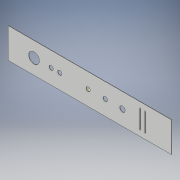
# Autodesk Inventor part: Faceplate
Saved by Autodesk Inventor 2017 (Build 210142000, 142)
## iProperties
Created: 2017-03-30
Part Number: Faceplate
Material: Generic
Document SubType Name: Sheet Metal
Designer: plumbj
Density: 1 g/cm^3
Appearance: Default
Sheet Metal Rule: Default
Author: plumbj
Autodesk Inventor part; units mm, degrees
ref_plane "YZ Plane" through (0, 0, 0) normal (1, 0, 0) x (0, 1, 0)
ref_plane "XZ Plane" through (0, 0, 0) normal (0, 1, 0) x (-1, 0, 0)
ref_plane "XY Plane" through (0, 0, 0) normal (0, 0, 1) x (1, 0, 0)
sketch "Sketch1" plane through (0, 0, 0) normal (0, 0, 1) x (1, 0, 0)
  line L0 (-241.3, -44.45) -> (241.3, -44.45)
  line L1 (241.3, -44.45) -> (241.3, 44.45)
  line L2 (241.3, 44.45) -> (-241.3, 44.45)
  line L3 (-241.3, 44.45) -> (-241.3, -44.45)
  point P0 (0, 0)
  dimension "d0" = 482.6
  dimension "d1" = 88.9
  dimension "d62" = 44.45
  dimension "d63" = 241.3
  constraints: 8 end point, 2 parallel, 1 horizontal, 1 perpendicular
  measures "d0" distance of L2.end L1.end
  measures "d1" distance of L1.end L0.end
  measures "d62" distance from line of L2 point (0, 0)
  measures "d63" distance from line of point (0, 0) L1
extrude "Extrusion1" add sketch "Sketch1" along normal blind 1.1113
sketch "Sketch3" plane through (0, 0, 1.1113) normal (0, 0, 1) x (1, 0, 0)
  point P0 (0, 0)
sketch "Sketch4" plane through (0, 0, 1.1113) normal (0, 0, 1) x (1, 0, 0)
  line L0 (147.5, 26.0031) -> (150.1, 26.0031)
  line L1 (150.1, 26.0031) -> (150.1, -25.9969)
  line L2 (150.1, -25.9969) -> (147.5, -25.9969)
  line L3 (147.5, -25.9969) -> (147.5, 26.0031)
  line L4 (162.5, 26.0031) -> (165.1, 26.0031)
  line L5 (165.1, 26.0031) -> (165.1, -25.9969)
  line L6 (165.1, -25.9969) -> (162.5, -25.9969)
  line L7 (162.5, -25.9969) -> (162.5, 26.0031)
  line L8 (-241.3, -44.45) -> (241.3, -44.45) projected
  line L9 (241.3, -44.45) -> (241.3, 44.45) projected
  circle A0 centre (-114.3, 0) radius 6.2484
  circle A1 centre (-88.9, 0) radius 6.2484
  circle A2 centre (-4.9, 0) radius 6.2484
  circle A3 centre (45.9, 0) radius 6.5
  circle A4 centre (96.7, 0) radius 8
  line L10 (241.3, 44.45) -> (-241.3, 44.45) projected
  line L11 (-241.3, -44.45) -> (241.3, -44.45) projected
  line L12 (241.3, -44.45) -> (241.3, 44.45) projected
  line L13 (241.3, 44.45) -> (-241.3, 44.45) projected
  line L14 (-241.3, 44.45) -> (-241.3, -44.45) projected
  circle A5 centre (163.8, 28.0031) radius 1.05
  circle A6 centre (163.8, -27.9969) radius 1.05
  circle A7 centre (148.8, 28.0031) radius 1.05
  circle A8 centre (148.8, -27.9969) radius 1.05
  circle A9 centre (-165.1, 0) radius 15.875
  point P0 (0, 0)
  dimension "d9" = 2.6
  dimension "d12" = 2.6
  dimension "d13" = 52
  dimension "d17" = 18.4531
  dimension "d18" = 52
  dimension "d20" = 18.4531
  dimension "d22" = 12.4968
  dimension "d23" = 12.4968
  dimension "d24" = 12.4968
  dimension "d26" = 13
  dimension "d27" = 16
  dimension "d28" = 50.8
  dimension "d35" = 44.45
  dimension "d36" = 44.45
  dimension "d38" = 44.45
  dimension "d40" = 44.45
  dimension "d42" = 50.8
  dimension "d47" = 2.1
  dimension "d48" = 2.1
  dimension "d49" = 56
  dimension "d50" = 2
  dimension "d51" = 1.3
  dimension "d52" = 1.3
  dimension "d53" = 2.1
  dimension "d54" = 2.1
  dimension "d55" = 56
  dimension "d56" = 1.3
  dimension "d57" = 1.3
  dimension "d58" = 2
  dimension "d59" = 76.2
  dimension "d65" = 31.75
  dimension "d66" = 25.4
  dimension "d67" = 44.45
  dimension "d68" = 50.8
  dimension "d69" = 76.2
  dimension "d70" = 44.45
  dimension "d71" = 50.8
  dimension "d74" = 15
  constraints: 16 end point, 10 centre point, 4 parallel, 2 horizontal, 2 perpendicular
  measures "d9" distance of L1.end L2.end
  measures "d12" distance of L5.end L6.end
  measures "d13" distance of L4.end L5.end
  measures "d17" distance between parallel lines of L8 L2
  measures "d18" distance between parallel lines of L2 L0
  measures "d20" distance between parallel lines of L8 L6
  measures "d22" diameter of A0
  measures "d23" diameter of A1
  measures "d24" diameter of A2
  measures "d26" diameter of A3
  measures "d27" diameter of A4
  measures "d28" distance from line of L3 A4.centre
  measures "d35" distance from line of L10 A3.centre
  measures "d36" distance from line of L10 A1.centre
  measures "d38" distance from line of L8 A0.centre
  measures "d40" distance from line of L8 A4.centre
  measures "d42" distance of A4.centre A3.centre
  measures "d47" diameter of A5
  measures "d48" diameter of A6
  measures "d49" distance of A5.centre A6.centre
  measures "d50" distance from line of L6 A6.centre
  measures "d51" distance from line of L7 A6.centre
  measures "d52" distance from line of L7 A5.centre
  measures "d53" diameter of A7
  measures "d54" diameter of A8
  measures "d55" distance of A7.centre A8.centre
  measures "d56" distance from line of L1 A8.centre
  measures "d57" distance from line of A7.centre L3
  measures "d58" distance from line of L2 A8.centre
  measures "d59" distance between parallel lines of L9 L5
  measures "d65" diameter of A9
  measures "d66" distance of A0.centre A1.centre
  measures "d67" distance from line of L13 A9.centre
  measures "d68" distance of A0.centre A9.centre
  measures "d69" distance from line of A9.centre L14
  measures "d70" distance from line of L10 A2.centre
  measures "d71" distance of A3.centre A2.centre
  measures "d74" distance of A5.centre A7.centre
extrude "Extrusion3" cut sketch "Sketch4" against normal up to next contours L0 L1 L2 L3 | L4 L5 L6 L7 | A0 | A1 | A2 | A3 | A4 | A5 | A6 | A7 | A8 | A9
body "Solid1"
